Supermicro SSD Mount (Autodesk Fusion 360 design; units mm, degrees)
Autodesk Fusion 360 part; units mm, degrees
ref_plane "WorkPlane1" through (0, 12, 0) normal (0, 1, 0) x (0, 0, 1)
sketch "Sketch1" plane through (0, 0, 0) normal (0, 1, 0) x (1, 0, 0)
  circle A0 centre (0, 0) radius 1.65
  circle A1 centre (0, 0) radius 4
  circle A2 centre (0, 77) radius 1.65
  circle A3 centre (0, 77) radius 4
  circle A4 centre (62, 0) radius 1.65
  circle A5 centre (62, 0) radius 4
  circle A6 centre (62, 77) radius 4
  circle A7 centre (62, 77) radius 1.65
  line L0 (-7, 84) -> (69, 84)
  line L1 (69, 84) -> (69, -7)
  line L2 (69, -7) -> (-7, -7)
  line L3 (-7, -7) -> (-7, 84)
  line L4 (4, 73) -> (58, 73)
  line L5 (58, 73) -> (58, 4)
  line L6 (58, 4) -> (4, 4)
  line L7 (4, 4) -> (4, 73)
  line L8 (-7, -52) -> (4, -52)
  line L9 (4, -52) -> (4, -7)
  line L10 (4, -7) -> (-7, -7)
  line L11 (-7, -7) -> (-7, -52)
  line L12 (69, -7) -> (58, -7)
  line L13 (58, -7) -> (58, -52)
  line L14 (58, -52) -> (69, -52)
  line L15 (69, -52) -> (69, -7)
  line L16 (-7, -20) -> (69, -20)
  line L17 (69, -20) -> (69, -52)
  line L18 (69, -52) -> (-7, -52)
  line L19 (-7, -52) -> (-7, -20)
  dimension "d1" = 3.3
  dimension "d2" = 8
  dimension "d3" = 3.3
  dimension "d4" = 8
  dimension "d5" = 77
  dimension "d6" = 3.3
  dimension "d7" = 8
  dimension "d8" = 62
  dimension "d9" = 3.3
  dimension "d10" = 8
  dimension "d11" = 77
  dimension "d12" = 7
  dimension "d13" = 7
  dimension "d14" = 7
  dimension "d15" = 7
  dimension "d16" = 4
  dimension "d17" = 4
  dimension "d18" = 4
  dimension "d19" = 4
  dimension "d52" = 45
  dimension "d53" = 11
  dimension "d54" = 45
  dimension "d55" = 11
  dimension "d65" = 20
  constraint coincident A0.centre A1.centre
  constraint concentric A0 A1
  constraint concentric A2 A3
  constraint concentric A4 A5
  constraint concentric A6 A7
  constraint horizontal A0.centre A4.centre
  constraint vertical A4.centre A6.centre
  constraint vertical A0.centre A2.centre
  constraint horizontal L0
  constraint vertical L1
  constraint horizontal L2
  constraint vertical L3
  constraint horizontal L4
  constraint vertical L5
  constraint horizontal L6
  constraint vertical L7
  constraint horizontal L8
  constraint vertical L9
  constraint horizontal L10
  constraint vertical L11
  constraint collinear L2 L10
  constraint horizontal L12
  constraint vertical L13
  constraint horizontal L14
  constraint vertical L15
  constraint horizontal L16
  constraint vertical L17
  constraint horizontal L18
  constraint vertical L19
  constraint coincident L11 L16.start
  measures "d1" diameter of A0
  measures "d2" diameter of A1
  measures "d3" diameter of A2
  measures "d4" diameter of A3
  measures "d5" distance of A0.centre A2.centre
  measures "d6" diameter of A4
  measures "d7" diameter of A5
  measures "d8" distance of A0.centre A4.centre
  measures "d9" diameter of A7
  measures "d10" diameter of A6
  measures "d11" distance of A4.centre A6.centre
  measures "d12" distance of A2.centre L3
  measures "d13" distance of A2.centre L0
  measures "d14" distance of A4.centre L1
  measures "d15" distance of A4.centre L2
  measures "d16" distance of A2.centre L7
  measures "d17" distance of A2.centre L4
  measures "d18" distance of A4.centre L5
  measures "d19" distance of A4.centre L6
  measures "d52" distance of L1.end L14.end
  measures "d53" distance of L13.end L14.end
  measures "d54" distance of L8.start L2.end
  measures "d55" distance of L8.start L8.end
  measures "d65" distance of A0.centre L16
extrude "Extrude1" add sketch "Sketch1" along normal blind 3 contours L0 L1 L2 L3 L10 L12 | L2 L9 L10 L11 L16 | L2 L12 L13 L15 L16 | L8 L9 L11 L16 L18 L19 | L13 L14 L15 L16 L17 L18
extrude "Extrude2" add sketch "Sketch1" along normal blind 2 contours A1 | A3 | A5 | A6
sketch "Sketch3" plane through (0, 0, 0) normal (1, 0, 0) x (0, 0, -1)
  circle A0 centre (32, 7) radius 1.65
  circle A1 centre (32, 7) radius 3.75
  line L0 (84, 0) -> (-52, 0)
  line L1 (77, 0) -> (32, 0)
  line L2 (39, 12) -> (25, 12)
  line L3 (25, 12) -> (25, 3)
  line L4 (25, 3) -> (39, 3)
  line L5 (39, 3) -> (39, 12)
  line L6 (4, 3) -> (73, 3)
  circle A2 centre (-45, 7) radius 1.65
  circle A3 centre (-45, 7) radius 3.75
  line L7 (32, 0) -> (-45, 0)
  line L8 (-38, 12) -> (-52, 12)
  line L9 (-52, 12) -> (-52, 0)
  line L10 (-52, 0) -> (-38, 0)
  line L11 (-38, 0) -> (-38, 12)
  line L12 (-7, 0) -> (-52, 0)
  point P0 (77, 0)
  dimension "d24" = 3.3
  dimension "d25" = 7.5
  dimension "d27" = 45
  dimension "d28" = 7
  dimension "d29" = 5
  dimension "d30" = 7
  dimension "d31" = 7
  dimension "d32" = 3.3
  dimension "d33" = 7.5
  dimension "d34" = 77
  dimension "d35" = 7
  dimension "d36" = 5
  dimension "d37" = 7
  dimension "d38" = 7
  constraint concentric A0 A1
  constraint coincident P0 L1.start
  constraint parallel L0 L1
  constraint horizontal L2
  constraint vertical L3
  constraint horizontal L4
  constraint vertical L5
  constraint vertical A0.centre L1.end
  constraint concentric A2 A3
  constraint parallel L1 L7
  constraint vertical A2.centre L7.end
  constraint horizontal L8
  constraint vertical L9
  constraint horizontal L10
  constraint vertical L11
  constraint coincident L4.end L6
  constraint coincident L10.end L12
  measures "d24" diameter of A0
  measures "d25" diameter of A1
  measures "d27" distance of P0 L1.end
  measures "d28" distance of A0.centre L1.end
  measures "d29" distance of A0.centre L2
  measures "d30" distance of A0.centre L5
  measures "d31" distance of A0.centre L3
  measures "d32" diameter of A2
  measures "d33" diameter of A3
  measures "d34" distance of L1.end L7.end
  measures "d35" distance of A2.centre L7.end
  measures "d36" distance of A2.centre L8
  measures "d37" distance of A2.centre L9
  measures "d38" distance of A2.centre L11
extrude "Extrude3" add sketch "Sketch3" along normal blind 3 from surface at -7 contours L0 L7 L8 L9 L10 L11 L12 | L2 L3 L4 L5 L6
extrude "Extrude5" add sketch "Sketch3" along normal blind 2 from surface at -6 contours A1 | A3
extrude "Extrude6" add sketch "Sketch3" along normal blind 3 from surface at 66 contours L0 L7 L8 L9 L10 L11 L12 | L2 L3 L4 L5 L6
extrude "Extrude7" add sketch "Sketch3" along normal blind 2 from surface at 66 contours A1 | A3
fillet "Fillet1" radius 4.5 4 edges at (-7, 1.5, -84) (69, 1.5, -84) (4, 1.5, 52) (58, 1.5, 52)
fillet "Fillet2" radius 4.5 6 edges at (4, 1.5, -73) (4, 1.5, -4) (58, 1.5, -4) (58, 1.5, -73) (4, 1.5, 7) (58, 1.5, 7)
extrude "Extrude8" cut sketch "Sketch1" along normal blind 1 contours L8 L9 L11 L16 L18 L19 | L13 L14 L15 L16 L17 L18 | L9 L13 L16 L18
fillet "Fillet3" radius 3.5 8 edges at (67.5, 12, -25) (-5.5, 12, -25) (-5.5, 12, 52) (-5.5, 12, 38) (67.5, 12, 52) (67.5, 12, 38) (67.5, 12, -39) (-5.5, 12, -39)
